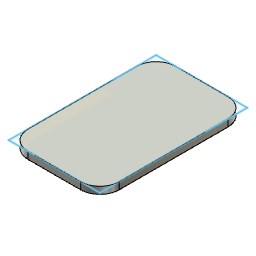
Holder (Autodesk Fusion 360 design; units mm, degrees)
Autodesk Fusion 360 part; units mm, degrees
sketch "sketch 317" plane through (0, 0, 0) normal (0, 0, 1) x (1, 0, 0)
  line L0 (110, 0) -> (-20, 0)
  line L1 (110, 210) -> (110, 0)
  line L2 (-20, 210) -> (110, 210)
  line L3 (-20, 0) -> (-20, 210)
extrude "Extrude1" add sketch "sketch 317" against normal blind 10
fillet "Fillet1" radius 27.5 4 edges at (110, 0, -5) (-20, 0, -5) (-20, 210, -5) (110, 210, -5)
